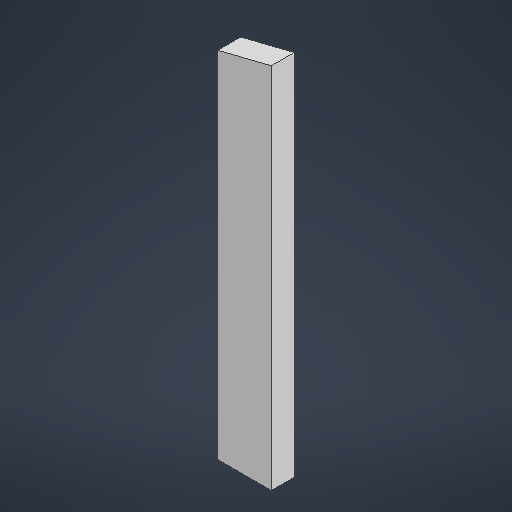
# Autodesk Inventor part: S2_2x4x24
Saved by Autodesk Inventor 2026 (Build 300175000, 175)
## iProperties
Created: 2025-09-04
Part Number: S2_2x4x24
Material: Generic
Document SubType Name: Modeling
Designer: trott
Density: 1 g/cm^3
Appearance: Default
Author: trott
Autodesk Inventor part; units mm, degrees
ref_plane "YZ Plane" through (0, 0, 0) normal (1, 0, 0) x (0, 1, 0)
ref_plane "XZ Plane" through (0, 0, 0) normal (0, 1, 0) x (-1, 0, 0)
ref_plane "XY Plane" through (0, 0, 0) normal (0, 0, 1) x (1, 0, 0)
sketch "Sketch1" plane through (0, 0, 0) normal (0, 0, 1) x (1, 0, 0)
  line L0 (0, 0) -> (1219.2, 0)
  line L1 (0, 0) -> (0, 1524)
  line L2 (0, 1524) -> (0, 1828.8)
  line L3 (0, 1524) -> (609.6, 1524)
  line L4 (609.6, 1524) -> (1219.2, 0)
  line L5 (0, 1828.8) -> (609.6, 1524)
  line L6 (609.6, 1524) -> (1219.2, 1524)
  line L7 (1219.2, 1524) -> (1219.2, 914.4)
  line L8 (1219.2, 914.4) -> (914.4, 914.4)
  line L9 (914.4, 914.4) -> (1219.2, 1524)
  line L10 (914.4, 914.4) -> (880.5333, 846.6667)
  line L11 (1219.2, 1524) -> (1219.2, 2133.6)
  line L12 (1219.2, 2133.6) -> (0, 1828.8)
  line L13 (880.5333, 846.6667) -> (801.0188, 886.424)
  line L14 (1219.2, 1524) -> (1139.6854, 1563.7573)
  line L15 (1139.6854, 1563.7573) -> (801.0188, 886.424)
  line L16 (1219.2, 1524) -> (1130.3, 1524)
  line L17 (1130.3, 1524) -> (1130.3, 2111.375)
  line L18 (1219.2, 2133.6) -> (1240.7614, 2047.3543)
  line L19 (0, 1828.8) -> (21.5614, 1742.5543)
  line L20 (21.5614, 1742.5543) -> (1240.7614, 2047.3543)
  point P0 (1119.8068, 1524)
  point P1 (836.3586, 957.1036)
  point P2 (1219.2, 2041.964)
  point P3 (1130.3, 2019.739)
  dimension "d21" = 1219.2
  dimension "d22" = 1524
  dimension "d23" = 304.8
  dimension "d24" = 609.6
  dimension "d25" = 609.6
  dimension "d26" = 609.6
  dimension "d27" = 304.8
  dimension "d28" = 609.6
  dimension "d29" = 88.9
  dimension "d30" = 88.9
  dimension "d31" = 90
  dimension "d32" = 90
  dimension "d33" = 88.9
  dimension "d34" = 88.9
  dimension "d35" = 88.9
  dimension "d36" = 90
  dimension "d37" = 90
  constraints: 42 end point, 7 point on line, 4 perpendicular, 2 horizontal, 1 vertical
  measures "d21" distance of L0.start L0.end
  measures "d22" distance of L0.start L1.end
  measures "d23" distance of L1.end L2.end
  measures "d24" distance of L1.end L3.end
  measures "d25" distance of L3.end L6.end
  measures "d26" distance of L6.end L7.end
  measures "d27" distance of L7.end L8.end
  measures "d28" distance of L6.end L11.end
  measures "d29" distance of L10.end L13.end
  measures "d30" distance of L6.end L14.end
  measures "d31" angle of L14 L9
  measures "d32" angle of L10 L13
  measures "d33" distance of L6.end L16.end
  measures "d34" distance of L11.end L18.end
  measures "d35" distance of L2.end L19.end
  measures "d36" angle of L12 L19
  measures "d37" angle of L12 L18
extrude "Extrusion2" add sketch "Sketch1" along normal blind 38.1 contours L12 L11 L20 L17 | L14 L15 L17 L20 L11 | L6 L17 L15 L14
body "Solid2"
